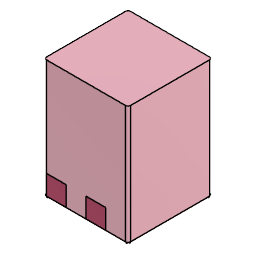
front_leg (Autodesk Fusion 360 design; units mm, degrees)
part number: 2025-09-29-17-41-02-140
Autodesk Fusion 360 part; units mm, degrees
sketch "Leg" plane through (0, 0, 0) normal (0, 0, 1) x (1, 0, 0)
  line L0 (0, 0) -> (67, 0)
  line L1 (67, 0) -> (67, 67)
  line L2 (67, 67) -> (0, 67)
  line L3 (0, 67) -> (0, 0)
  dimension "d2" = 67
  dimension "d3" = 67
  constraint horizontal L0
  constraint vertical L1
  constraint horizontal L2
  constraint vertical L3
  constraint coincident L0.start L3.end
  measures "d2" distance of L0.start L0.end
  measures "d3" distance of L0.end L1.end
extrude "Extrude1" add sketch "Leg" along normal blind 96 makes body 1
sketch "Toes" plane through (0, 0, 0) normal (0, -1, 0) x (1, 0, 0)
  line L0 (0, 0) -> (67, 0)
  line L1 (67, 0) -> (67, 96)
  line L2 (67, 96) -> (0, 96)
  line L3 (0, 96) -> (0, 0)
  line L4 (2, 17.75) -> (17.75, 17.75)
  line L5 (17.75, 17.75) -> (17.75, 2)
  line L6 (17.75, 2) -> (2, 2)
  line L7 (2, 2) -> (2, 17.75)
  line L8 (33.5, 17.75) -> (49.25, 17.75)
  line L9 (49.25, 17.75) -> (49.25, 2)
  line L10 (49.25, 2) -> (33.5, 2)
  line L11 (33.5, 2) -> (33.5, 17.75)
  dimension "d16" = 15.75
  dimension "d17" = 15.75
  dimension "d18" = 15.75
  dimension "d19" = 2
  dimension "d20" = 2
  dimension "d21" = 15.75
  dimension "d22" = 17.75
  constraint horizontal L4
  constraint vertical L5
  constraint horizontal L6
  constraint vertical L7
  constraint horizontal L8
  constraint vertical L9
  constraint horizontal L10
  constraint vertical L11
  constraint collinear L6 L10
  constraint collinear L4 L8
  measures "d16" distance of L5.end L6.end
  measures "d17" distance of L9.end L10.end
  measures "d18" distance of L5 L11
  measures "d19" distance of L3 L7
  measures "d20" distance of L0 L6
  measures "d21" distance of L4.start L6.end
  measures "d22" distance of L1 L9
extrude "Extrude3" add sketch "Toes" along normal blind 0.01 separate body contours L4 L5 L6 L7 | L8 L9 L10 L11 makes body 2 at (7.25, 0, 7.25) makes body 3 at (38.75, 0, 7.25)
fillet "Fillet1" radius 2 8 edges at (0, 67, 48) (0, 33.5, 0) (0, 0, 48) (33.5, 0, 0) (67, 0, 48) (33.5, 67, 0) (67, 33.5, 0) (67, 67, 48) on bodies 1
equation "leg_width = 67 mm" comment "The dimensions of the 67 mm x 67 mm pine post used for the Legs."
equation "d2 = leg_width"
equation "d3 = leg_width"
equation "block_size = 16 mm" comment "The size of the blocks used for the dimensions of the Minecraft Pig."
equation "d5 = leg_height"
equation "fillet_radius = 2 mm" comment "The radius of the fillets applied to the Legs."
equation "d16 = toe_width"
equation "d17 = toe_width"
equation "d18 = toe_width"
equation "d19 = fillet_radius"
equation "d20 = fillet_radius"
equation "d21 = toe_width"
equation "d26 = fillet_radius"
equation "toe_width = ( leg_width - 2 * fillet_radius ) / 4" comment "The width and height of the two toes."
equation "leg_height = 6 * block_size" comment "The height of the Minecraft Pig's Legs."
named bodies: "Front Leg", "Right Toe", "Left Toe"
